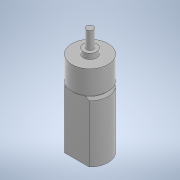
# Autodesk Inventor part: Motor
Saved by Autodesk Inventor 2022 (Build 260153000, 153)
## iProperties
Created: 2022-08-09
Part Number: Motor
Material: Generic
Document SubType Name: Modeling
Designer: Nick
Density: 4.1256 g/cm^3
Appearance: Smooth - Medium Gray
Mass: 28 g
Surface Area: 23.5381 cm^2
Volume: 6.7869 cm^3
Author: Nick
Autodesk Inventor part; units mm, degrees
ref_plane "YZ Plane" through (0, 0, 0) normal (1, 0, 0) x (0, 1, 0)
ref_plane "XZ Plane" through (0, 0, 0) normal (0, 1, 0) x (-1, 0, 0)
ref_plane "XY Plane" through (0, 0, 0) normal (0, 0, 1) x (1, 0, 0)
sketch "Sketch6" plane through (0, 0, 0) normal (0, 0, 1) x (1, 0, 0)
  line L0 (0, 0) -> (8, 0)
  line L1 (8, 0) -> (8, 37.56)
  line L2 (8, 37.56) -> (0, 37.56)
  line L3 (0, 37.56) -> (0, 0)
  line L4 (0, 37.56) -> (1.5, 37.56)
  line L5 (1.5, 37.56) -> (1.5, 47.59)
  line L6 (1.5, 47.59) -> (0, 47.59)
  line L7 (0, 47.59) -> (0, 37.56)
  line L8 (8, 27.3) -> (7, 26.3)
  line L9 (7, 26.3) -> (8, 25.3)
  line L10 (1.5, 37.56) -> (2.975, 37.56)
  line L11 (2.975, 37.56) -> (2.975, 39.94)
  line L12 (2.975, 39.94) -> (1.5, 39.94)
  line L13 (1.5, 39.94) -> (1.5, 37.56)
  dimension "d31" = 16
  dimension "d32" = 3
  dimension "d35" = 1
  dimension "d36" = 11.26
  dimension "d38" = 26.3
  dimension "d39" = 2.38
  dimension "d40" = 5.95
  dimension "d41" = 7.65
  constraints: 28 end point, 6 parallel, 5 perpendicular, 3 horizontal, 2 point on line
  measures "d31" diameter of L1 L3
  measures "d32" diameter of L5 L7
  measures "d35" distance from line of L1 L8.end
  measures "d36" distance from line of L2 L8.end
  measures "d38" distance from line of L0 L8.end
  measures "d39" distance of L10.end L11.end
  measures "d40" diameter of L11 L7
  measures "d41" distance between parallel lines of L12 L6
revolve "Revolution2" add sketch "Sketch6" angle 360 about axis through (0, 37.56, 0) along (0, -1, 0) contours L3 L2 L1 L8 L9 L0 | L7 L6 L5 L2 | L5 L12 L11 L2
sketch "Sketch7" plane through (0, 0, 0) normal (0, -1, 0) x (1, 0, 0)
  line L0 (-5.4569, 8) -> (5.4569, 8)
  line L1 (5.4569, 8) -> (5.4569, 5.85)
  line L2 (5.4569, 5.85) -> (-5.4569, 5.85)
  line L3 (-5.4569, 5.85) -> (-5.4569, 8)
  line L4 (5.4569, -8) -> (-5.4569, -8)
  line L5 (-5.4569, -8) -> (-5.4569, -5.85)
  line L6 (-5.4569, -5.85) -> (5.4569, -5.85)
  line L7 (5.4569, -5.85) -> (5.4569, -8)
  circle A0 centre (0, 0) radius 8 projected
  dimension "d42" = 11.7
  constraints: 16 end point, 4 parallel, 4 point on circle, 2 horizontal, 2 perpendicular, 2 tangent, 1 collinear
  measures "d42" distance between parallel lines of L6 L2
extrude "Extrusion5" cut sketch "Sketch7" against normal blind 26.3 contours L0 A0 L3 | L0 L1 A0 | A0 L2 | L6 A0
body "Solid2"
